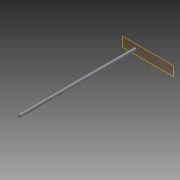
# Autodesk Inventor part: Part18
Saved by Autodesk Inventor 2015 (Build 190159000, 159)
## iProperties
Created: 2014-10-18
Part Number: Part18
Material: Generic
Document SubType Name: Modeling
Designer: jesse
Density: 1 g/cm^3
Appearance: Default
Author: jesse
Autodesk Inventor part; units mm, degrees
ref_plane "YZ Plane" through (0, 0, 0) normal (1, 0, 0) x (0, 1, 0)
ref_plane "XZ Plane" through (0, 0, 0) normal (0, 1, 0) x (-1, 0, 0)
ref_plane "XY Plane" through (0, 0, 0) normal (0, 0, 1) x (1, 0, 0)
ref_plane "Work Plane1" through (0, 0, 0) normal (0, 0, 1) x (1, 0, 0)
sketch "Sketch1" plane through (0, 0, 0) normal (0, 0, 1) x (1, 0, 0)
  circle A0 centre (93.0941, -9.525) radius 3.175 projected
  line L0 (0, 0) -> (0, -19.05) projected
  line L1 (0, -19.05) -> (101.6, -19.05) projected
  line L2 (101.6, 0) -> (101.6, -19.05) projected
  line L3 (0, 0) -> (101.6, 0) projected
  line L4 (31.1152, -67.3136) -> (74.0512, -63.5572) projected
  line L5 (17.5579, 87.6465) -> (31.1152, -67.3136) projected
  line L6 (60.4939, 91.403) -> (17.5579, 87.6465) projected
  line L7 (26.8927, -19.05) -> (25.226, 0)
  circle A1 centre (22.8843, -9.525) radius 3.175
  line L8 (74.0512, -63.5572) -> (60.4939, 91.403) projected
  constraints: 4 point on line, 2 end point, 1 centre point
extrude "Extrusion1" add sketch "Sketch1" along normal blind 254 contours A1 L5 | L5 A1
body "Solid1"
